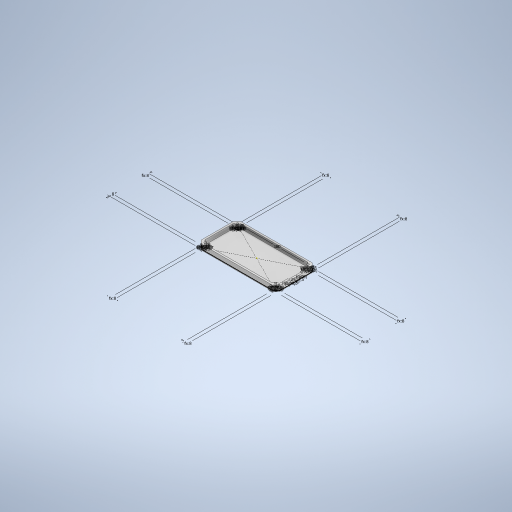
# Autodesk Inventor part: enclosed base
Saved by Autodesk Inventor 2023 (Build 270158000, 158)
## iProperties
Created: 2022-05-30
Part Number: enclosed base
Material: Generic
Document SubType Name: Modeling
Designer: Aakif
Density: 1 g/cm^3
Appearance: Default
Author: Aakif
Autodesk Inventor part; units mm, degrees
ref_plane "YZ Plane" through (0, 0, 0) normal (1, 0, 0) x (0, 1, 0)
ref_plane "XZ Plane" through (0, 0, 0) normal (0, 1, 0) x (-1, 0, 0)
ref_plane "XY Plane" through (0, 0, 0) normal (0, 0, 1) x (1, 0, 0)
sketch "Sketch1" plane through (0, 0, 0) normal (0, 1, 0) x (-1, 0, 0)
  line L0 (82, 45) -> (-82, 45)
  line L1 (-90, 37) -> (-90, -37)
  line L2 (-82, -45) -> (82, -45)
  line L3 (90, -37) -> (90, 37)
  line L4 (90, 45) -> (-90, -45) construction
  line L5 (-90, 45) -> (90, -45) construction
  line L6 (90, 37) -> (82, 45)
  line L7 (90, -37) -> (82, -45)
  line L8 (-82, 45) -> (-90, 37)
  line L9 (-82, -45) -> (-90, -37)
  line L10 (90, -37) -> (80.892, -37)
  line L11 (80.892, -37) -> (80.892, -37.187)
  line L12 (80.892, -37) -> (81.079, -37) construction
  circle A0 centre (80.892, -37.187) radius 0.725
  circle A1 centre (80.892, -37.187) radius 2.225
  line L13 (90, 37) -> (80.892, 37)
  line L14 (80.892, 37) -> (80.892, 37.187)
  circle A2 centre (80.892, 37.187) radius 0.725
  circle A3 centre (80.892, 37.187) radius 2.225
  line L15 (-90, 37) -> (-80.892, 37)
  line L16 (-90, 37) -> (-80.892, 37) construction
  line L17 (-80.892, 37) -> (-80.892, 37.187)
  circle A4 centre (-80.892, 37.187) radius 0.725
  circle A5 centre (-80.892, 37.187) radius 2.225
  line L18 (-90, -37) -> (-80.892, -37)
  line L19 (-90, -37) -> (-80.892, -37) construction
  line L20 (-80.892, -37) -> (-80.892, -37.187)
  line L21 (-80.892, -37) -> (-80.705, -37) construction
  circle A6 centre (-80.892, -37.187) radius 0.725
  circle A7 centre (-80.892, -37.187) radius 2.225
  line L22 (80.892, -37.187) -> (80.892, -34.287)
  line L23 (80.892, -37.187) -> (83.792, -37.187) construction
  line L24 (80.892, -37.187) -> (77.992, -37.187)
  line L25 (80.892, -37.187) -> (83.792, -37.187) construction
  line L26 (77.992, -37.187) -> (77.992, -45)
  line L27 (80.892, 37.187) -> (80.892, 34.287)
  line L28 (80.892, 37.187) -> (83.792, 37.187) construction
  line L29 (80.892, 34.287) -> (90, 34.287)
  line L30 (80.892, 37.187) -> (77.992, 37.187)
  line L31 (80.892, 37.187) -> (83.792, 37.187) construction
  line L32 (-80.892, -37.187) -> (-80.892, -34.287)
  line L33 (-80.892, -37.187) -> (-77.992, -37.187) construction
  line L34 (-80.892, -34.287) -> (-90, -34.287)
  line L35 (-80.892, -37.187) -> (-77.992, -37.187)
  line L36 (-80.892, -37.187) -> (-77.992, -37.187) construction
  line L37 (-77.992, -37.187) -> (-77.992, -45)
  line L38 (-77.992, -37.187) -> (-70.179, -37.187) construction
  line L39 (-80.892, 37.187) -> (-77.992, 37.187)
  line L40 (-80.892, 37.187) -> (-77.992, 37.187) construction
  line L41 (-77.992, 37.187) -> (-77.992, 45)
  line L42 (-80.892, 37.187) -> (-80.892, 34.287)
  line L43 (-80.892, 37.187) -> (-77.992, 37.187) construction
  line L44 (-80.892, 34.287) -> (-90, 34.287)
  line L45 (-77.992, 37.187) -> (-77.992, 34.287)
  line L46 (-77.992, 34.287) -> (-80.892, 34.287)
  line L47 (-80.892, -34.287) -> (-77.992, -34.287)
  line L48 (-77.992, -34.287) -> (-77.992, -37.187)
  line L49 (77.992, 37.187) -> (77.992, 45)
  line L50 (77.992, 37.187) -> (85.805, 37.187) construction
  line L51 (80.892, 34.287) -> (77.992, 34.287)
  line L52 (77.992, 34.287) -> (77.992, 37.187)
  line L53 (80.892, -34.287) -> (90, -34.287)
  line L54 (80.892, -34.287) -> (90, -34.287) construction
  line L55 (77.992, -37.187) -> (77.992, -34.287)
  line L56 (77.992, -34.287) -> (80.892, -34.287)
  line L57 (-90, 0) -> (-90, 14.5)
  line L58 (-90, 0) -> (-90, -14.5)
  line L59 (-90, -14.5) -> (-86, -14.5)
  line L60 (-90, -14.5) -> (-86, -14.5) construction
  line L61 (-86, -14.5) -> (-86, 14.5)
  line L62 (-86, 14.5) -> (-90, 14.5)
  point P0 (0, 0)
  point P1 (-90, -34.287)
  point P2 (77.992, -45)
  point P3 (90, -34.287)
  point P4 (90, 34.287)
  point P5 (-90, 34.287)
  dimension "d31" = 12
  dimension "d0" = 180
  dimension "d1" = 90
  dimension "d2" = 8
  dimension "d3" = 8
  dimension "d4" = 8
  dimension "d5" = 8
  dimension "d6" = 8
  dimension "d7" = 8
  dimension "d8" = 8
  dimension "d9" = 8
  dimension "d34" = 9.108
  dimension "d35" = 0.187
  dimension "d36" = 90
  dimension "d37" = 1.45
  dimension "d38" = 4.45
  dimension "d39" = 9.108
  dimension "d40" = 0.187
  dimension "d41" = 90
  dimension "d42" = 1.45
  dimension "d43" = 4.45
  dimension "d44" = 9.108
  dimension "d45" = 0
  dimension "d46" = 0.187
  dimension "d47" = 90
  dimension "d48" = 1.45
  dimension "d49" = 4.45
  dimension "d50" = 9.108
  dimension "d51" = 0
  dimension "d52" = 0.187
  dimension "d53" = 90
  dimension "d54" = 1.45
  dimension "d55" = 4.45
  dimension "d58" = 2.9
  dimension "d59" = 90
  dimension "d62" = 2.9
  dimension "d63" = 180
  dimension "d64" = 7.813
  dimension "d65" = 90
  dimension "d66" = 2.9
  dimension "d67" = 90
  dimension "d68" = 9.108
  dimension "d69" = 90
  dimension "d70" = 2.9
  dimension "d71" = 180
  dimension "d74" = 2.9
  dimension "d75" = 90
  dimension "d76" = 9.108
  dimension "d77" = 90
  dimension "d78" = 2.9
  dimension "d79" = 0
  dimension "d80" = 7.813
  dimension "d81" = 90
  dimension "d82" = 2.9
  dimension "d83" = 0
  dimension "d84" = 7.813
  dimension "d85" = 90
  dimension "d86" = 2.9
  dimension "d87" = 90
  dimension "d88" = 9.108
  dimension "d89" = 90
  dimension "d90" = 2.9
  dimension "d91" = 2.9
  dimension "d92" = 2.9
  dimension "d93" = 2.9
  constraints: 126 end point, 27 horizontal, 19 equal length, 13 perpendicular, 10 point on line, 8 centre point, 8 coincident, 7 vertical, 3 midpoint
  measures "d0" distance of L5.end L4.end
  measures "d1" distance of L4.end L5.start
  measures "d2" distance of L3.end L4.start
  measures "d3" distance of L0.start L4.start
  measures "d4" distance of L3.start L5.end
  measures "d5" distance of L2.end L5.end
  measures "d6" distance of L0.end L5.start
  measures "d7" distance of L1.start L5.start
  measures "d8" distance of L2.start L4.end
  measures "d9" distance of L1.end L4.end
  measures "d34" distance of L3.start L10.end
  measures "d35" distance of L10.end L11.end
  measures "d36" angle of L11 L12
  measures "d37" diameter of A0
  measures "d38" diameter of A1
  measures "d39" distance of L3.end L13.end
  measures "d40" distance of L13.end L14.end
  measures "d41" angle of L13 L14
  measures "d42" diameter of A2
  measures "d43" diameter of A3
  measures "d44" distance of L1.start L15.end
  measures "d45" distance between parallel lines of L15 L16
  measures "d46" distance of L15.end L17.end
  measures "d47" angle of L17 L15
  measures "d48" diameter of A4
  measures "d49" diameter of A5
  measures "d50" distance of L1.end L18.end
  measures "d51" distance between parallel lines of L18 L19
  measures "d52" distance of L19.end L20.end
  measures "d53" angle of L20 L21
  measures "d54" diameter of A6
  measures "d55" diameter of A7
  measures "d58" distance of L22.start L22.end
  measures "d59" angle of L23 L22
  measures "d62" distance of L22.start L24.end
  measures "d63" angle of L24 L25
  measures "d64" distance of L24.end L26.end
  measures "d65" angle of L26 L24
  measures "d66" distance of L27.start L27.end
  measures "d67" angle of L27 L28
  measures "d68" distance of L27.end L29.end
  measures "d69" angle of L29 L27
  measures "d70" distance of L27.start L30.end
  measures "d71" angle of L30 L31
  measures "d74" distance of L32.start L32.end
  measures "d75" angle of L33 L32
  measures "d76" distance of L32.end L34.end
  measures "d77" angle of L34 L32
  measures "d78" distance of L32.start L33.end
  measures "d79" distance between parallel lines of L35 L36
  measures "d80" distance of L36.end L37.end
  measures "d81" angle of L37 L38
  measures "d82" distance of L39.start L39.end
  measures "d83" distance between parallel lines of L39 L40
  measures "d84" distance of L39.end L41.end
  measures "d85" angle of L41 L39
  measures "d86" distance of L39.start L42.end
  measures "d87" angle of L42 L43
  measures "d88" distance of L42.end L44.end
  measures "d89" angle of L42 L44
  measures "d90" distance of L43.end L45.end
  measures "d91" distance of L45.end L42.end
  measures "d92" distance of L32.end L47.end
  measures "d93" distance of L47.end L36.end
extrude "Extrusion1" add sketch "Sketch1" against normal blind 2
sketch "Sketch2" plane through (0, 0, 0) normal (0, 1, 0) x (1, 0, 0)
  line L0 (-82, -45) -> (82, -45)
  line L1 (90, -37) -> (90, 37)
  line L2 (82, 45) -> (-82, 45)
  line L3 (-90, 37) -> (-90, -37)
  line L4 (-90, -45) -> (90, 45) construction
  line L5 (90, -45) -> (-90, 45) construction
  line L6 (-90, -37) -> (-82, -45)
  line L7 (-90, 37) -> (-82, 45)
  line L8 (82, 45) -> (90, 37)
  line L9 (82, -45) -> (90, -37)
  line L10 (-86, -35.3431) -> (-80.3431, -41)
  line L11 (-80.3431, -41) -> (80.3431, -41)
  line L12 (80.3431, -41) -> (86, -35.3431)
  line L13 (86, -35.3431) -> (86, 35.3431)
  line L14 (86, 35.3431) -> (80.3431, 41)
  line L15 (80.3431, 41) -> (-80.3431, 41)
  line L16 (-80.3431, 41) -> (-86, 35.3431)
  line L17 (-86, 35.3431) -> (-86, -35.3431)
  line L18 (0, 0) -> (90, 0)
  line L19 (90, 0) -> (90, -14.5)
  line L20 (90, -14.5) -> (0, -14.5)
  line L21 (0, -14.5) -> (0, 0)
  line L22 (0, 0) -> (90, 0)
  line L23 (90, 0) -> (90, 14.5)
  line L24 (90, 14.5) -> (0, 14.5)
  line L25 (0, 14.5) -> (0, 0)
  line L26 (-90, 35) -> (-81.5147, 26.5147)
  circle A0 centre (-81.5147, 26.5147) radius 1.45
  circle A1 centre (-81.5147, 26.5147) radius 4.45
  line L27 (-90, 35) -> (-77.0647, 35)
  line L28 (-77.0647, 35) -> (-77.0647, 22.0647)
  line L29 (-77.0647, 22.0647) -> (-90, 22.0647)
  line L30 (-90, 22.0647) -> (-90, 35)
  circle A2 centre (-81.5147, -26.5147) radius 1.45
  circle A3 centre (-81.5147, -26.5147) radius 4.45
  line L31 (-90, -35) -> (-77.0647, -35)
  line L32 (-77.0647, -35) -> (-77.0647, -22.0647)
  line L33 (-77.0647, -22.0647) -> (-90, -22.0647)
  line L34 (-90, -22.0647) -> (-90, -35)
  circle A4 centre (81.5147, 26.5147) radius 1.45
  circle A5 centre (81.5147, 26.5147) radius 4.45
  line L35 (77.0647, 35) -> (77.0647, 22.0647)
  line L36 (77.0647, 22.0647) -> (90, 22.0647)
  line L37 (77.0647, -22.0647) -> (90, -22.0647)
  line L38 (77.0647, -35) -> (77.0647, -22.0647)
  circle A6 centre (81.5147, -26.5147) radius 4.45
  circle A7 centre (81.5147, -26.5147) radius 1.45
  line L39 (90, -35) -> (77.0647, -35)
  line L40 (90, -22.0647) -> (90, -35)
  point P0 (86, -14.5)
  point P1 (86, 14.5)
  point P2 (81.5147, 22.0647)
  point P3 (86, 22.0647)
  point P4 (77.0647, 31)
  point P5 (77.0647, 26.5147)
  point P6 (77.0647, -26.5147)
  point P7 (77.0647, -31)
  point P8 (86, -22.0647)
  point P9 (81.5147, -22.0647)
  point P10 (-77.0647, -26.5147)
  point P11 (-81.5147, -22.0647)
  point P12 (-86, -22.0647)
  point P13 (-77.0647, -31)
  point P14 (-86, 22.0647)
  point P15 (-81.5147, 22.0647)
  point P16 (-77.0647, 26.5147)
  point P17 (-77.0647, 31)
  dimension "d12" = 180
  dimension "d13" = 90
  dimension "d14" = 8
  dimension "d15" = 8
  dimension "d16" = 8
  dimension "d17" = 8
  dimension "d18" = 8
  dimension "d19" = 8
  dimension "d20" = 8
  dimension "d21" = 8
  dimension "d22" = 4
  dimension "d23" = 90
  dimension "d24" = 14.5
  dimension "d25" = 90
  dimension "d26" = 14.5
  dimension "d31" = 12
  dimension "d32" = 2.9
  dimension "d33" = 3
  constraints: 82 end point, 14 symmetric about line, 10 parallel, 8 centre point, 8 point on line, 5 perpendicular, 4 horizontal, 2 midpoint, 1 coincident, 13 other
  measures "d12" distance of L5.end L4.end
  measures "d13" distance of L4.end L5.start
  measures "d14" distance of L3.end L4.start
  measures "d15" distance of L0.start L4.start
  measures "d16" distance of L3.start L5.end
  measures "d17" distance of L2.end L5.end
  measures "d18" distance of L2.start L4.end
  measures "d19" distance of L1.end L4.end
  measures "d20" distance of L0.end L5.start
  measures "d21" distance of L1.start L5.start
  measures "d22" distance between parallel lines of L3 L17
  measures "d23" distance of L19.end L20.end
  measures "d24" distance of L18.end L19.end
  measures "d25" distance of L24.end L23.end
  measures "d26" distance of L23.end L22.end
  measures "d31" distance of L26.start L26.end
  measures "d32" diameter of A0
  measures "d33" radial gap between concentric circles of A0 A1
extrude "Extrusion4" add sketch "Sketch2" along normal blind 10 contours L6 L3 L31 L17 L10 L11 L12 L13 L39 L1 L9 L0 | L3 L33 L17 L31 | L39 L13 L37 L1 | L3 L29 L17 L33 | L37 L13 L20 L1 | L3 L26 L17 L29 | L27 L17 L26 | L3 L7 L2 L8 L1 L36 L13 L14 L15 L16 L17 L27 | L24 L13 L36 L1
extrude "Extrusion5" add sketch "Sketch1" along normal blind 10 contours L6 L13 A3 L30 L49 L0 | L3 L29 L27 A3 L13 | L41 L39 A5 L15 L8 L0 | L30 A3 L27 L51 L52 | L45 L46 L42 A5 L39 | L3 L10 A1 L22 L53 | L15 A5 L42 L44 L1 | L7 L2 L26 L24 A1 L10 | L22 A1 L24 L55 L56 | L2 L9 L18 A7 L35 L37 | L35 A7 L32 L47 L48 | L34 L32 A7 L18 L1
extrude "Extrusion6" add sketch "Sketch1" along normal blind 8 contours L62 L61 L59 L1
fillet "Fillet1" radius 3 12 edges at (-77.992, 5, -41) (-77.992, 5, -34.287) (-86, 5, -34.287) (86, 5, -34.287) (77.992, 5, -34.287) (77.992, 5, -41) (86, 5, 34.287) (77.992, 5, 34.287) (77.992, 5, 41) (-77.992, 5, 34.287) (-86, 5, 34.287) (-77.992, 5, 41)
equation "\"d3\" = d2"
equation "\"d4\" = d2"
equation "\"d5\" = d4"
equation "\"d6\" = d2"
equation "\"d7\" = d6"
equation "\"d8\" = d2"
equation "\"d9\" = d8"
equation "\"d15\" = d14"
equation "\"d16\" = d14"
equation "\"d17\" = d16"
equation "\"d18\" = d14"
equation "\"d19\" = d18"
equation "\"d20\" = d14"
equation "\"d21\" = d20"
body "Solid1"
